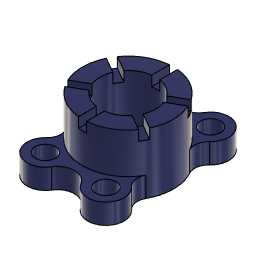
mechanial_body v1 (Autodesk Fusion 360 design; units mm, degrees)
Autodesk Fusion 360 part; units mm, degrees
note: some values were not read from the file. Set by a fixed rule: which sketch regions a step uses.
sketch "Sketch1" plane through (0, 0, 0) normal (0, 0, 1) x (1, 0, 0)
  circle A0 centre (0, 0) radius 275
  circle A1 centre (0, 0) radius 450
  line L0 (0, 0) -> (0, 1300) construction
  line L1 (0, 0) -> (1400, 0) construction
  line L2 (0, 0) -> (-820.061, 1420.3873) construction
  circle A2 centre (-300, 519.6152) radius 100
  circle A3 centre (300, 519.6152) radius 100
  arc A4 (-145.7143, 612.3294) -> (145.7143, 612.3294) centre (0, 699.8928) ccw
  arc A5 (-394.2776, 216.899) -> (-422.0297, 387.2946) centre (-516.9418, 284.3786) ccw
  arc A6 (422.0297, 387.2946) -> (394.2776, 216.899) centre (516.9418, 284.3786) ccw
  arc A7 (-145.7143, 612.3294) -> (-422.0297, 387.2946) centre (-300, 519.6152) ccw
  arc A8 (422.0297, 387.2946) -> (145.7143, 612.3294) centre (300, 519.6152) ccw
  arc A9 (-422.0297, -387.2946) -> (-394.2776, -216.899) centre (-516.9418, -284.3786) ccw
  arc A10 (-422.0297, -387.2946) -> (-145.7143, -612.3294) centre (-300, -519.6152) ccw
  arc A11 (145.7143, -612.3294) -> (-145.7143, -612.3294) centre (0, -699.8928) ccw
  arc A12 (145.7143, -612.3294) -> (422.0297, -387.2946) centre (300, -519.6152) ccw
  arc A13 (394.2776, -216.899) -> (422.0297, -387.2946) centre (516.9418, -284.3786) ccw
  circle A14 centre (-300, -519.6152) radius 100
  circle A15 centre (300, -519.6152) radius 100
  dimension "d1" = 550
  dimension "d2" = 900
  dimension "d3" = 30
  dimension "d4" = 200
  dimension "d5" = 360
  dimension "d6" = 600
  dimension "d7" = 170
  dimension "d8" = 140
  constraint coincident A0.centre A1.centre
  constraint concentric A0 A1
  constraint vertical L0
  constraint perpendicular L0 L1
  constraint coincident L2 A2.centre
  constraint concentric A2 A7
  constraint symmetric L0 A2 A3
  constraint symmetric L0 A7 A8
  constraint tangent A4 A8
  constraint tangent A1 A5
  constraint coincident A1 A5.start
  constraint tangent A4 A7
  constraint tangent A5 A7
  constraint symmetric L0 A5.end A6.start
  constraint symmetric L0 A5.start A6.end
  constraint symmetric L0 A5 A6
  constraint symmetric L1 A2 A14
  constraint symmetric L1 A3 A15
  constraint symmetric L1 A4.start A10.end
  constraint symmetric L1 A4.end A11.start
  constraint symmetric L1 A4 A11
  constraint symmetric L1 A5.end A9.start
  constraint symmetric L1 A5.start A9.end
  constraint symmetric L1 A5 A9
  constraint symmetric L1 A6.end A13.start
  constraint symmetric L1 A6.start A12.end
  constraint symmetric L1 A6 A13
  constraint symmetric L1 A7 A10
  constraint symmetric L1 A8 A12
  measures "d1" diameter of A0
  measures "d2" diameter of A1
  measures "d3" angle of L0 L2
  measures "d4" diameter of A2
  measures "d5" diameter of A7
  measures "d6" distance of A0.centre A2.centre
  measures "d7" radius of A4
  measures "d8" radius of A5
extrude "Extrude1" add sketch "Sketch1" along normal blind 200 contours A1 A4 A5 A6 A7 A8 | A1 A9 A10 A11 A12 A13 makes body 1 at (-383.5434, 235.3603, 133.3333) makes body 2 at (383.5434, -235.3603, 133.3333)
extrude "Extrude2" add sketch "Sketch1" along normal blind 600 contours A1 bodies 1 2
sketch "Sketch2" plane through (0, 0, 600) normal (0, 0, 1) x (-1, 0, 0)
  circle A0 centre (0, 0) radius 275
  circle A1 centre (0, 0) radius 450
  line L0 (37.0395, -264.2232) -> (-42.9605, -264.2232)
  line L1 (-42.9605, -264.2232) -> (-42.9605, -454.2232)
  line L2 (-42.9605, -454.2232) -> (37.0395, -454.2232)
  line L3 (37.0395, -454.2232) -> (37.0395, -264.2232)
  line L4 (37.0395, -264.2232) -> (-42.9605, -454.2232) construction
  line L5 (-42.9605, -264.2232) -> (37.0395, -454.2232) construction
  point P0 (-2.9605, -359.2232)
  dimension "d13" = 80
  dimension "d14" = 190
  constraint horizontal L0
  constraint perpendicular L0 L1
  constraint parallel L0 L2
  constraint parallel L1 L3
  constraint coincident L4 P0
  constraint coincident L5 P0
  measures "d13" distance of L1.end L2.end
  measures "d14" distance of L0.end L1.end
extrude "Extrude3" cut sketch "Sketch2" against normal blind 100 contours A0 A1 L1 L3 picked at (28.1553, -331.9237) bodies 1
pattern_circular "C-Pattern1" count 6 over 360 about axis through (0, 0, 600) along (0, 0, 1) of "Extrude3"
